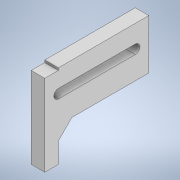
# Autodesk Inventor part: Encoder_Mount3_Base
Saved by Autodesk Inventor 2022 (Build 260153000, 153)
## iProperties
Created: 2024-04-30
Part Number: Encoder_Mount3_Base
Material: Generic
Document SubType Name: Modeling
Designer: Gotham City
Density: 1 g/cm^3
Appearance: Default
Author: Gotham City
Autodesk Inventor part; units mm, degrees
ref_plane "YZ Plane" through (0, 0, 0) normal (1, 0, 0) x (0, 1, 0)
ref_plane "XZ Plane" through (0, 0, 0) normal (0, 1, 0) x (-1, 0, 0)
ref_plane "XY Plane" through (0, 0, 0) normal (0, 0, 1) x (1, 0, 0)
sketch "Sketch1" plane through (0, 0, 0) normal (0, 0, 1) x (1, 0, 0)
  line L0 (-19.3, -12.5) -> (26, -12.5)
  line L1 (26, -12.5) -> (26, 12.5)
  line L2 (26, 12.5) -> (-19.3, 12.5)
  line L3 (-19.3, 12.5) -> (-19.3, -12.5)
  line L4 (-36.76, 0) -> (36.46, 0) construction
  line L5 (-9, -12.5) -> (-9, 12.5) construction
  circle A0 centre (0, 0) radius 9 construction
  line L6 (-22.8, -12.5) -> (-22.8, 12.5) construction
  line L7 (-26.3, -12.5) -> (-19.3, -12.5) construction
  line L8 (-19.3, -12.5) -> (-19.3, 12.5) construction
  line L9 (-19.3, 12.5) -> (-26.3, 12.5) construction
  line L10 (-26.3, 12.5) -> (-26.3, -12.5) construction
  dimension "d0" = 25
  dimension "d1" = 35
  dimension "d2" = 13.8
  dimension "d3" = 7
  constraints: 20 end point, 7 point on line, 4 parallel, 4 perpendicular, 2 horizontal, 1 tangent, 2 other
  measures "d0" distance of L2.end L0.start
  measures "d1" distance between parallel lines of L1 L5
  measures "d2" distance between parallel lines of L5 L6
  measures "d3" distance between parallel lines of L8 L10
extrude "Extrusion1" add sketch "Sketch1" along normal blind 3
sketch "Sketch2" plane through (0, 0, 0) normal (0, 0, -1) x (-1, 0, 0)
  line L0 (-26, -12.5) -> (-26, 12.5) projected
  line L1 (-26, 12.5) -> (19.3, 12.5) projected
  line L2 (-26, -12.5) -> (-21.5, -12.5)
  line L3 (-21.5, -12.5) -> (-21.5, 12.5)
  line L4 (-21.5, 12.5) -> (-26, 12.5)
  line L5 (-26, 12.5) -> (-26, -12.5)
  point P0 (0, 0)
  dimension "d6" = 4.5
  constraints: 8 end point, 2 parallel, 1 horizontal, 1 perpendicular, 1 point on line
  measures "d6" distance between parallel lines of L0 L3
extrude "Extrusion2" add sketch "Sketch2" along normal blind 8
sketch "Sketch3" plane through (21.5, -12.5, 0) normal (-1, 0, 0) x (0, 0, 1)
  line L0 (-8, 25) -> (3, 25) construction
  line L1 (3, 0) -> (-8, 0) construction
  line L2 (0, 25) -> (-8, 0) construction
  point P0 (0, 12.5)
  point P1 (-4, 12.5)
  constraints: 2 end point, 1 midpoint, 1 point on line
hole "Hole1" at (21.5, 0, -4) direction (1, 0, 0) diameter 2.6 end through all clearance for "Socket Head Cap Screw ISO 4762" size "M2.5" standard "ISO"
sketch "Sketch4" plane through (21.5, -12.5, 0) normal (-1, 0, 0) x (0, 0, 1)
  circle A0 centre (-4, 12.5) radius 1.3 projected
  line L0 (-2.4123, 15.25) -> (-0.8246, 12.5)
  line L1 (-0.8246, 12.5) -> (-2.4123, 9.75)
  line L2 (-2.4123, 9.75) -> (-5.5877, 9.75)
  line L3 (-5.5877, 9.75) -> (-7.1754, 12.5)
  line L4 (-7.1754, 12.5) -> (-5.5877, 15.25)
  line L5 (-5.5877, 15.25) -> (-2.4123, 15.25)
  point P0 (0, 12.5)
  dimension "d16" = 5.5
  constraints: 12 end point, 1 coincident, 1 horizontal, 13 other
  measures "d16" distance between parallel lines of L2 L5
extrude "Extrusion3" cut sketch "Sketch4" against normal blind 2.5
fillet "Fillet2" radius 7 1 edges at (-19.3, 12.5, 1.5)
sketch "Sketch5" plane through (0, 0, 0) normal (0, 0, -1) x (-1, 0, 0)
  line L0 (2, 0) -> (-2, 0) construction
  line L1 (2, 1.3) -> (-2, 1.3)
  line L2 (-2, -1.3) -> (2, -1.3)
  arc A0 (2, -1.3) -> (2, 1.3) centre (2, 0) ccw
  arc A1 (-2, 1.3) -> (-2, -1.3) centre (-2, 0) ccw
  point P0 (0, 0)
  dimension "d19" = 2.6
  dimension "d20" = 4
  constraints: 8 end point, 4 point on circle, 4 tangent, 2 centre point, 1 horizontal, 1 midpoint, 1 parallel
  measures "d19" distance between parallel lines of L2 L1
  measures "d20" distance of L0.start L0.end
extrude "Extrusion4" cut sketch "Sketch5" against normal through all
sketch "Sketch7" plane through (0, 0, 0) normal (0, 0, -1) x (-1, 0, 0)
  line L0 (19.3, 12.5) -> (19.3, -12.5) projected
  line L1 (19.3, -12.5) -> (-26, -12.5) projected
  line L2 (19.3, 12.5) -> (15.3, 12.5)
  line L3 (15.3, 12.5) -> (15.3, -12.5)
  line L4 (15.3, -12.5) -> (19.3, -12.5)
  line L5 (19.3, -12.5) -> (19.3, 12.5)
  line L6 (19.3, 12.5) -> (19.3, -12.5) projected
  line L7 (19.3, 6) -> (15.3, 6)
  line L8 (15.3, 6) -> (15.3, -5)
  line L9 (15.3, -5) -> (19.3, -5)
  line L10 (19.3, -5) -> (19.3, 6)
  line L11 (-35.06, 0) -> (28.36, 0) construction
  point P0 (0, 0)
  dimension "d23" = 4
  dimension "d25" = 11
  dimension "d26" = 6
  constraints: 16 end point, 4 parallel, 3 point on line, 2 horizontal, 2 perpendicular
  measures "d23" distance between parallel lines of L0 L3
  measures "d25" distance between parallel lines of L9 L7
  measures "d26" distance between parallel lines of L11 L7
extrude "Extrusion5" add sketch "Sketch7" along normal blind 20 contours L0 L9 L3 L7
chamfer "Chamfer1" distance 3 angle 45 2 edges at (-15.3, 0.5, 0) (21.5, 0, 0)
chamfer "Chamfer2" distance 3 angle 45 2 edges at (-15.7911, 6, 0) (-15.8, -5, 0)
sketch "Sketch9" plane through (0, 0, -20) normal (0, 0, -1) x (-1, 0, 0)
  line L0 (18.1161, -1) -> (16.4661, -1)
  line L1 (16.4661, -1) -> (16.4661, 3.1)
  line L2 (16.4661, 3.1) -> (18.1161, 3.1)
  line L3 (18.1161, 3.1) -> (18.1161, -1)
  line L4 (19.3, 6) -> (15.3, 6) projected
  line L5 (15.3, 6) -> (19.2821, 6) projected
  line L6 (17.2911, 6) -> (17.2911, 3.1) construction
  point P0 (0, 0)
  dimension "d37" = 7
  dimension "d38" = 4.1
  dimension "d39" = 1.65
  constraints: 10 end point, 2 midpoint, 2 parallel, 1 horizontal, 1 perpendicular, 1 vertical
  measures "d37" distance between parallel lines of L0 L4
  measures "d38" distance of L2.end L0.start
  measures "d39" distance between parallel lines of L1 L3
extrude "Extrusion6" cut sketch "Sketch9" against normal through all
sketch "Sketch10" plane through (-19.3, -12.5, 0) normal (-1, 0, 0) x (0, 0, 1)
  line L0 (-20, 15.6) -> (-20, 11.5) construction
  line L1 (-20, 13.55) -> (3.0284, 13.55) construction
  line L2 (-17, 13.55) -> (0, 13.55) construction
  line L3 (-17, 12.55) -> (0, 12.55)
  line L4 (0, 14.55) -> (-17, 14.55)
  arc A0 (-17, 14.55) -> (-17, 12.55) centre (-17, 13.55) ccw
  arc A1 (0, 12.55) -> (0, 14.55) centre (0, 13.55) ccw
  line L5 (3, 18) -> (3, 0) projected
  point P0 (0, 12.5)
  point P1 (-8.5, 13.55)
  dimension "d42" = 2
  dimension "d43" = 3
  dimension "d44" = 3
  constraints: 10 end point, 4 point on circle, 4 tangent, 2 centre point, 2 midpoint, 2 point on line, 1 horizontal, 1 parallel
  measures "d42" distance between parallel lines of L4 L3
  measures "d43" distance from line of L0 L2.start
  measures "d44" distance from line of L5 L2.end
extrude "Extrusion7" cut sketch "Sketch10" against normal up to next
sketch "Sketch11" plane through (-19.3, -12.5, 0) normal (-1, 0, 0) x (0, 0, 1)
  line L0 (-17, 14.55) -> (0, 14.55) projected
  arc A0 (0, 12.55) -> (0, 14.55) centre (0, 13.55) ccw projected
  line L1 (0, 12.55) -> (-17, 12.55) projected
  arc A1 (-17, 14.55) -> (-17, 12.55) centre (-17, 13.55) ccw projected
  line L2 (0, 18) -> (3, 18) projected
  line L3 (0, 18) -> (0, 18.5) projected
  line L4 (0, 18.5) -> (-20, 18.5) projected
  line L5 (-20, 7.5) -> (-20, 18.5) projected
  line L6 (-3, 7.5) -> (-20, 7.5) projected
  line L7 (0, 4.5) -> (-3, 7.5) projected
  line L8 (0, 4.5) -> (0, 0) projected
  line L9 (0, 0) -> (3, 0) projected
  line L10 (3, 18) -> (3, 0) projected
  point P0 (0, 12.5)
extrude "Extrusion8" add sketch "Sketch11" along normal blind 3 separate body
equation "\"d44\" = d43"
body "Solid1"
body "Solid2"
